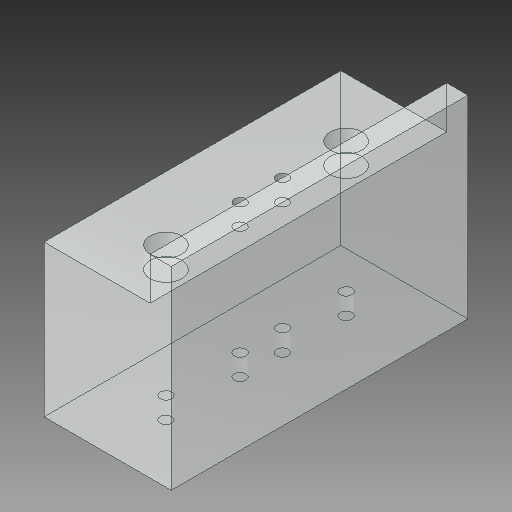
# Autodesk Inventor part: TSV-Support
Saved by Autodesk Inventor 2017 (Build 210142000, 142)
## iProperties
Created: 2017-03-27
Part Number: TSV-Support
Material: Generic
Document SubType Name: Modeling
Designer: hoeflinc
Density: 1 g/cm^3
Appearance: Clear
Author: hoeflinc
Autodesk Inventor part; units mm, degrees
ref_plane "YZ Plane" through (0, 0, 0) normal (1, 0, 0) x (0, 1, 0)
ref_plane "XZ Plane" through (0, 0, 0) normal (0, 1, 0) x (-1, 0, 0)
ref_plane "XY Plane" through (0, 0, 0) normal (0, 0, 1) x (1, 0, 0)
sketch "Sketch1" plane through (0, 0, 0) normal (0, 1, 0) x (-1, 0, 0)
  line L0 (0, 0) -> (38.1, 0)
  line L1 (38.1, 0) -> (38.1, -88.9)
  line L2 (38.1, -88.9) -> (0, -88.9)
  line L3 (0, -88.9) -> (0, 0)
  dimension "d0" = 88.9
  dimension "d1" = 38.1
  constraints: 8 end point, 2 parallel, 1 horizontal, 1 perpendicular
  measures "d0" distance of L2.end L0.start
  measures "d1" distance of L0.start L0.end
extrude "Extrusion1" add sketch "Sketch1" along normal blind 58.0644
sketch "Sketch6" plane through (0, 58.0644, 0) normal (0, 1, 0) x (1, 0, 0)
  line L0 (-38.1, 0) -> (0, 0) projected
  line L1 (0, 0) -> (0, 88.9) projected
  line L2 (0, 88.9) -> (-38.1, 88.9) projected
  line L3 (-38.1, 88.9) -> (-38.1, 0) projected
  line L4 (-38.1, 0) -> (-6.35, 0)
  line L5 (-6.35, 0) -> (-6.35, 88.9)
  line L6 (-6.35, 88.9) -> (-38.1, 88.9)
  line L7 (-38.1, 88.9) -> (-38.1, 0)
  dimension "d38" = 0
  dimension "d39" = 31.75
  dimension "d40" = 0
  dimension "d41" = 88.9
  constraints: 8 end point, 2 parallel, 1 horizontal, 1 perpendicular
  measures "d38" distance between parallel lines of L3 L7
  measures "d39" distance of L5.end L6.end
  measures "d40" distance between parallel lines of L2 L6
  measures "d41" distance of L4.end L5.end
extrude "Extrusion5" cut sketch "Sketch6" against normal blind 12.7 contours L3 L2 L5 L0
sketch "Sketch7" plane through (0, 45.3644, 0) normal (0, 1, 0) x (1, 0, 0)
  arc A0 (-20.2095, 23.7057) -> (-20.2095, 11.2193) centre (-19.05, 17.4625) ccw projected
  line L0 (-26.5557, 23.7057) -> (-20.2095, 23.7057) projected
  line L1 (-26.5557, 11.2193) -> (-26.5557, 23.7057) projected
  line L2 (-26.5557, 11.2193) -> (-20.2095, 11.2193) projected
  arc A1 (-17.8905, 11.2193) -> (-17.8905, 23.7057) centre (-19.05, 17.4625) ccw projected
  line L3 (-17.8905, 11.2193) -> (-11.5443, 11.2193) projected
  line L4 (-11.5443, 23.7057) -> (-11.5443, 11.2193) projected
  line L5 (-17.8905, 23.7057) -> (-11.5443, 23.7057) projected
  arc A2 (-25.2932, 70.278) -> (-12.8068, 70.278) centre (-19.05, 71.4375) ccw projected
  line L6 (-25.2932, 70.278) -> (-25.2932, 63.9318) projected
  line L7 (-12.8068, 63.9318) -> (-25.2932, 63.9318) projected
  line L8 (-12.8068, 70.278) -> (-12.8068, 63.9318) projected
  arc A3 (-12.8068, 72.597) -> (-25.2932, 72.597) centre (-19.05, 71.4375) ccw projected
  line L9 (-12.8068, 78.9432) -> (-12.8068, 72.597) projected
  line L10 (-25.2932, 78.9432) -> (-12.8068, 78.9432) projected
  line L11 (-25.2932, 78.9432) -> (-25.2932, 72.597) projected
  circle A4 centre (-19.05, 52.3875) radius 1.7526 projected
  circle A5 centre (-19.05, 39.6875) radius 1.7526 projected
  point P0 (0, 0)
  constraints: 2 coincident
hole "Hole2" at (-19.05, 45.3644, -71.4375) at (-19.05, 45.3644, -17.4625) direction (0, -1, 0) diameter 9.525 depth 6.35 tip angle 118
sketch "Sketch8" plane through (0, 45.3644, 0) normal (0, 1, 0) x (1, 0, 0)
  circle A0 centre (-19.05, 52.3875) radius 1.7526 projected
  circle A1 centre (-19.05, 39.6875) radius 1.7526 projected
  point P0 (0, 0)
  constraints: 2 coincident
hole "Hole3" at (-19.05, 45.3644, -52.3875) at (-19.05, 45.3644, -39.6875) direction (0, -1, 0) diameter 3.5052 depth 6.35 tip angle 118
sketch "Sketch9" plane through (0, 0, 0) normal (0, -1, 0) x (1, 0, 0)
  line L0 (0, 0) -> (-38.1, 0) projected
  line L1 (-38.1, 0) -> (-38.1, -88.9) projected
  line L2 (-38.1, -88.9) -> (0, -88.9) projected
  line L3 (0, -88.9) -> (0, 0) projected
  circle A0 centre (-19.05, -17.4625) radius 4.7625 projected
  circle A1 centre (-19.05, -71.4375) radius 4.7625 projected
  circle A2 centre (-19.05, -39.6875) radius 1.7526 projected
  circle A3 centre (-19.05, -52.3875) radius 1.7526 projected
  circle A4 centre (-19.05, -39.6875) radius 1.7526 projected
  circle A5 centre (-19.05, -52.3875) radius 1.7526 projected
  constraints: 4 coincident
hole "Hole4" at (-19.05, 0, -17.4625) at (-19.05, 0, -71.4375) at (-19.05, 0, -39.6875) at (-19.05, 0, -52.3875) direction (0, 1, 0) diameter 3.5052 depth 6.35 tip angle 118
thread "Thread1" size "6-32 UNC" class "2B" standard "ANSI Unified Screw Threads" full length
thread "Thread2" size "6-32 UNC" class "2B" standard "ANSI Unified Screw Threads" full length
thread "Thread3" size "6-32 UNC" class "2B" standard "ANSI Unified Screw Threads" full length
thread "Thread4" size "6-32 UNC" class "2B" standard "ANSI Unified Screw Threads" full length
thread "Thread5" size "6-32 UNC" class "2B" standard "ANSI Unified Screw Threads" full length
thread "Thread6" size "6-32 UNC" class "2B" standard "ANSI Unified Screw Threads" full length
body "Solid1"
